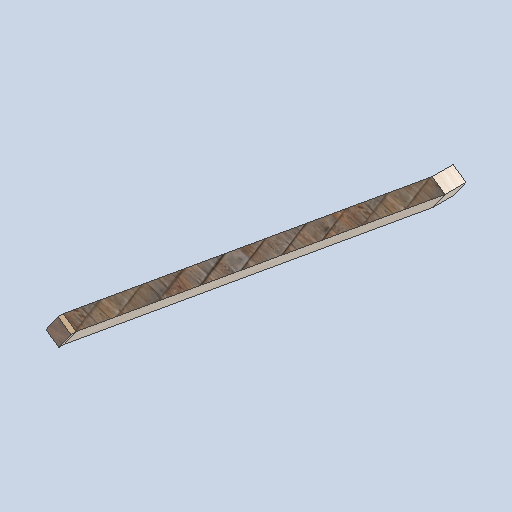
# Autodesk Inventor part: support_beam_segment_0102
Saved by Autodesk Inventor 2024.2 (Build 282272000, 272)
## iProperties
Created: 2024-05-20
Part Number: support_beam_segment_0102
Material: Wood Shake
Document SubType Name: Modeling
Designer: LOSTER_1
Density: 0.4 g/cm^3
Appearance: Shake - Handsplit
Author: LOSTER_1
Autodesk Inventor part; units mm, degrees
ref_plane "YZ Plane" through (0, 0, 0) normal (1, 0, 0) x (0, 1, 0)
ref_plane "XZ Plane" through (0, 0, 0) normal (0, 1, 0) x (-1, 0, 0)
sketch "Sketch1" plane through (0, 0, 0) normal (0, 0, 1) x (1, 0, 0)
  line L0 (-119.8302, -299.9423) -> (-234.5454, -463.7727)
  line L1 (3.0426, -385.9788) -> (-119.8302, -299.9423)
  line L2 (-111.6726, -549.8092) -> (3.0426, -385.9788)
  line L3 (-234.5454, -463.7727) -> (-111.6726, -549.8092)
  point P0 (0, 0)
  constraints: 8 end point
ref_plane "Work Plane2" through (0, 0, 3749) normal (0, 0, 1) x (1, 0, 0)
ref_plane "Work Plane1" through (0, 0, 0) normal (0, 0, 1) x (1, 0, 0)
sketch "Sketch2" plane through (0, 0, 3749) normal (0, 0, 1) x (1, 0, 0)
  line L0 (110.2028, 557.0196) -> (-4.5125, 393.1892) projected
  line L1 (233.0756, 470.9832) -> (110.2028, 557.0196) projected
  line L2 (118.3603, 307.1528) -> (233.0756, 470.9832) projected
  line L3 (-4.5125, 393.1892) -> (118.3603, 307.1528) projected
  point P0 (0, 0)
loft "Loft1" add profiles "Sketch1", "Sketch2"
sketch "Sketch3" plane through (0, 0, 0) normal (0, 0, 1) x (1, 0, 0)
  line L0 (-119.8302, -299.9423) -> (-234.5454, -463.7727) projected
  line L1 (3.0426, -385.9788) -> (-119.8302, -299.9423) projected
  line L2 (-111.6726, -549.8092) -> (3.0426, -385.9788) projected
  line L3 (-234.5454, -463.7727) -> (-111.6726, -549.8092) projected
  point P0 (0, 0)
sketch "Sketch4" plane through (-4.5125, 393.1892, 3749) normal (0, 0, 1) x (0.8192, -0.5736, 0)
  line L0 (0, 200) -> (0, 0) projected
  line L1 (0, 0) -> (150, 0) projected
  line L2 (150, 0) -> (150, 200) projected
  line L3 (150, 200) -> (0, 200) projected
  point P0 (229.2205, -319.4935)
extrude "Extrusion1" add sketch "Sketch3" against normal blind 200
extrude "Extrusion2" add sketch "Sketch4" along normal blind 50
body "Solid1"
